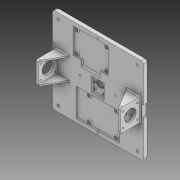
# Autodesk Inventor part: Topper
Saved by Autodesk Inventor 2020 (Build 240168000, 168)
## iProperties
Created: 2020-10-19
Part Number: Topper
Material: Generic
Document SubType Name: Modeling
Designer: DDeGo
Density: 1 g/cm^3
Appearance: Default
Author: DDeGo
Autodesk Inventor part; units mm, degrees
ref_plane "YZ Plane" through (0, 0, 0) normal (1, 0, 0) x (0, 1, 0)
ref_plane "XZ Plane" through (0, 0, 0) normal (0, 1, 0) x (-1, 0, 0)
sketch "Block1" plane through (0, 0, 0) normal (0, 0, 1) x (1, 0, 0)
  line L0 (-86.5, 19) -> (-20, 19) construction
  line L1 (-20, 19) -> (-20, 73.8) construction
  line L2 (-20, 73.8) -> (-86.5, 73.8) construction
  line L3 (-86.5, 73.8) -> (-86.5, 19) construction
  line L4 (-86.5, 19) -> (-20, 73.8) construction
  line L5 (-20, 19) -> (-86.5, 73.8) construction
  line L6 (-83, 22.15) -> (-23.5, 22.15) construction
  line L7 (-23.5, 22.15) -> (-23.5, 70.65) construction
  line L8 (-23.5, 70.65) -> (-83, 70.65) construction
  line L9 (-83, 70.65) -> (-83, 22.15) construction
  line L10 (-83, 22.15) -> (-23.5, 70.65) construction
  line L11 (-23.5, 22.15) -> (-83, 70.65) construction
  circle A0 centre (-23.5, 70.65) radius 1.35
  circle A1 centre (-83, 70.65) radius 1.35
  circle A2 centre (-23.5, 22.15) radius 1.35
  circle A3 centre (-83, 35) radius 1.35
  point P0 (-53.8698, 46.6979)
  point P1 (-53.25, 46.4)
  point P2 (-53.25, 46.4)
  dimension "d79" = 59.5
  dimension "d80" = 66.5
  dimension "d81" = 54.8
  dimension "d82" = 48.5
  dimension "d83" = 16
  dimension "d84" = 2.7
  measures "d79" distance of L7.end L8.end
  measures "d80" distance of L1.end L2.end
  measures "d81" distance of L0.end L1.end
  measures "d82" distance of L6.end L7.end
  measures "d83" distance from line of L0 A3.centre
  measures "d84" diameter of A3
sketch "Sketch1" plane through (0, 0, 0) normal (0, 0, 1) x (1, 0, 0)
  line L0 (-97.5, -92.5) -> (97.5, -92.5)
  line L1 (97.5, -92.5) -> (97.5, 92.5)
  line L2 (97.5, 92.5) -> (-97.5, 92.5)
  line L3 (-97.5, 92.5) -> (-97.5, -92.5)
  line L4 (-97.5, -92.5) -> (97.5, 92.5) construction
  line L5 (97.5, -92.5) -> (-97.5, 92.5) construction
  line L6 (85, -80) -> (-85, -80) construction
  line L7 (-85, -80) -> (-85, 80) construction
  line L8 (-85, 80) -> (85, 80) construction
  line L9 (85, 80) -> (85, -80) construction
  line L10 (85, -80) -> (-85, 80) construction
  line L11 (-85, -80) -> (85, 80) construction
  line L12 (-95.15, 90.15) -> (-74.85, 90.15)
  line L13 (-74.85, 90.15) -> (-74.85, 69.85)
  line L14 (-74.85, 69.85) -> (-95.15, 69.85)
  line L15 (-95.15, 69.85) -> (-95.15, 90.15)
  line L16 (-95.15, 90.15) -> (-74.85, 69.85) construction
  line L17 (-74.85, 90.15) -> (-95.15, 69.85) construction
  line L18 (95.15, 90.15) -> (74.85, 90.15)
  line L19 (74.85, 90.15) -> (74.85, 69.85)
  line L20 (74.85, 69.85) -> (95.15, 69.85)
  line L21 (95.15, 69.85) -> (95.15, 90.15)
  line L22 (95.15, 90.15) -> (74.85, 69.85) construction
  line L23 (74.85, 90.15) -> (95.15, 69.85) construction
  line L24 (95.15, -90.15) -> (74.85, -90.15)
  line L25 (74.85, -90.15) -> (74.85, -69.85)
  line L26 (74.85, -69.85) -> (95.15, -69.85)
  line L27 (95.15, -69.85) -> (95.15, -90.15)
  line L28 (95.15, -90.15) -> (74.85, -69.85) construction
  line L29 (74.85, -90.15) -> (95.15, -69.85) construction
  line L30 (-95.15, -90.15) -> (-74.85, -90.15)
  line L31 (-74.85, -90.15) -> (-74.85, -69.85)
  line L32 (-74.85, -69.85) -> (-95.15, -69.85)
  line L33 (-95.15, -69.85) -> (-95.15, -90.15)
  line L34 (-95.15, -90.15) -> (-74.85, -69.85) construction
  line L35 (-74.85, -90.15) -> (-95.15, -69.85) construction
  point P0 (0, 0)
  dimension "d0" = 195
  dimension "d2" = 170
  dimension "d23" = 185
  dimension "d24" = 160
  dimension "d113" = 20.3
  dimension "d114" = 20.3
  constraints: 72 end point, 12 midpoint, 12 parallel, 6 equal length, 6 horizontal, 6 perpendicular, 1 point on line
  measures "d0" distance of L1.end L2.end
  measures "d2" distance of L7.end L8.end
  measures "d23" distance of L0.end L1.end
  measures "d24" distance of L6.end L7.end
  measures "d113" distance of L12.start L12.end
  measures "d114" distance of L14.end L12.start
extrude "Extrusion1" add sketch "Sketch1" along normal blind 4
sketch "Sketch2" plane through (0, 0, 4) normal (0, 0, 1) x (1, 0, 0)
  line L0 (97.5, 92.5) -> (-97.5, 92.5) projected
  line L1 (97.5, -92.5) -> (-97.5, -92.5)
  line L2 (-97.5, -92.5) -> (-97.5, 92.5)
  line L3 (-97.5, 92.5) -> (97.5, 92.5)
  line L4 (97.5, 92.5) -> (97.5, -92.5)
  line L5 (97.5, -92.5) -> (-97.5, 92.5) construction
  line L6 (-97.5, -92.5) -> (97.5, 92.5) construction
  line L7 (-74.85, 69.85) -> (-95.15, 69.85) construction
  line L8 (-74.85, 90.15) -> (-74.85, 69.85) construction
  line L9 (-95.15, 69.85) -> (-74.85, 90.15) construction
  line L10 (74.85, 90.15) -> (95.15, 90.15) projected
  line L11 (95.15, 69.85) -> (74.85, 69.85) construction
  line L12 (74.85, 90.15) -> (95.15, 69.85) construction
  line L13 (74.85, -69.85) -> (95.15, -69.85) construction
  line L14 (74.85, -90.15) -> (74.85, -69.85) construction
  line L15 (95.15, -69.85) -> (74.85, -90.15) construction
  line L16 (-74.85, -90.15) -> (-95.15, -90.15) construction
  line L17 (-95.15, -90.15) -> (-95.15, -69.85) projected
  line L18 (-74.85, -90.15) -> (-95.15, -69.85) construction
  circle A0 centre (-85, 80) radius 2.75
  circle A1 centre (85, 80) radius 2.75
  circle A2 centre (85, -80) radius 2.75
  circle A3 centre (-85, -80) radius 2.75
  point P0 (0, 0)
  dimension "d7" = 5.5
  constraints: 16 end point, 4 centre point, 4 midpoint, 3 equal radius, 2 parallel, 1 horizontal, 1 perpendicular, 8 other
  measures "d7" diameter of A0
extrude "Extrusion2" add sketch "Sketch2" along normal blind 4
sketch "Sketch3" plane through (0, 0, 8) normal (0, 0, 1) x (1, 0, 0)
  line L0 (0, 0) -> (-96, 0) construction
  line L1 (0, 0) -> (96, 0) construction
  line L2 (-97.5, -12.5) -> (-94.5, -12.5)
  line L3 (-94.5, -12.5) -> (-94.5, 12.5)
  line L4 (-94.5, 12.5) -> (-97.5, 12.5)
  line L5 (-97.5, 12.5) -> (-97.5, -12.5)
  line L6 (-97.5, -12.5) -> (-94.5, 12.5) construction
  line L7 (-94.5, -12.5) -> (-97.5, 12.5) construction
  line L8 (94.5, -12.5) -> (97.5, -12.5)
  line L9 (97.5, -12.5) -> (97.5, 12.5)
  line L10 (97.5, 12.5) -> (94.5, 12.5)
  line L11 (94.5, 12.5) -> (94.5, -12.5)
  line L12 (94.5, -12.5) -> (97.5, 12.5) construction
  line L13 (97.5, -12.5) -> (94.5, 12.5) construction
  circle A0 centre (-85, 80) radius 2.75 projected
  line L14 (-85, 80) -> (-96, 0) construction
  circle A1 centre (85, 80) radius 2.75 projected
  line L15 (-97.5, 92.5) -> (-97.5, -92.5) projected
  dimension "d8" = 3
  dimension "d9" = 25
  constraints: 30 end point, 4 horizontal, 4 midpoint, 4 parallel, 3 equal length, 2 perpendicular, 1 point on line
  measures "d8" distance of L3.end L4.end
  measures "d9" distance of L2.end L3.end
extrude "Extrusion3" cut sketch "Sketch3" against normal through all contours L5 L4 L3 L2 | L11 L10 L9 L8
sketch "Sketch4" plane through (0, 0, 8) normal (0, 0, 1) x (1, 0, 0)
  line L0 (0, 0) -> (88.5, 0) construction
  line L1 (0, 0) -> (-88.5, 0) construction
  line L2 (-90.5, -21.15) -> (-86.5, -21.15)
  line L3 (-86.5, -21.15) -> (-86.5, 21.15)
  line L4 (-86.5, 21.15) -> (-90.5, 21.15)
  line L5 (-90.5, 21.15) -> (-90.5, -21.15)
  line L6 (-90.5, -21.15) -> (-86.5, 21.15) construction
  line L7 (-86.5, -21.15) -> (-90.5, 21.15) construction
  line L8 (86.5, -21.15) -> (90.5, -21.15)
  line L9 (90.5, -21.15) -> (90.5, 21.15)
  line L10 (90.5, 21.15) -> (86.5, 21.15)
  line L11 (86.5, 21.15) -> (86.5, -21.15)
  line L12 (86.5, -21.15) -> (90.5, 21.15) construction
  line L13 (90.5, -21.15) -> (86.5, 21.15) construction
  line L14 (-94.5, 12.5) -> (-94.5, -12.5) projected
  dimension "d13" = 42.3
  dimension "d14" = 4
  dimension "d22" = 8
  constraints: 28 end point, 4 horizontal, 4 midpoint, 4 parallel, 2 collinear, 2 perpendicular, 1 point on line
  measures "d13" distance of L2.end L3.end
  measures "d14" distance of L3.end L4.end
  measures "d22" distance between parallel lines of L14 L3
extrude "Extrusion4" add sketch "Sketch4" along normal blind 42.3
sketch "Sketch5" plane through (-90.5, -21.15, 8) normal (-1, 0, 0) x (0, 0, 1)
  line L0 (0, 0) -> (0, 42.3) projected
  line L1 (0, 0) -> (42.3, 0) projected
  line L2 (42.3, 42.3) -> (42.3, 0) projected
  line L3 (0, 42.3) -> (42.3, 42.3) projected
  line L4 (36.65, 5.65) -> (5.65, 5.65) construction
  line L5 (5.65, 5.65) -> (5.65, 36.65) construction
  line L6 (5.65, 36.65) -> (36.65, 36.65) construction
  line L7 (36.65, 36.65) -> (36.65, 5.65) construction
  line L8 (36.65, 36.65) -> (5.65, 5.65) construction
  circle A0 centre (36.65, 36.65) radius 1.75
  circle A1 centre (36.65, 5.65) radius 1.75
  circle A2 centre (21.15, 21.15) radius 12.5
  circle A3 centre (5.65, 5.65) radius 1.75
  circle A4 centre (5.65, 36.65) radius 1.75
  point P0 (-8, 21.15)
  dimension "d17" = 31
  dimension "d18" = 3.5
  dimension "d19" = 25
  constraints: 10 end point, 5 centre point, 4 coincident, 3 equal radius, 1 midpoint, 3 other
  measures "d17" distance of L6.end L4.start
  measures "d18" diameter of A1
  measures "d19" diameter of A2
extrude "Extrusion5" cut sketch "Sketch5" against normal through all contours A0 | A1 | A2 | A3 | A4
sketch "Sketch8" plane through (-90.5, -21.15, 8) normal (0, -1, 0) x (1, 0, 0)
  line L0 (4, 0) -> (0, 0) projected
  line L1 (4, 0) -> (4, 42.3) construction
  line L2 (0, 42.3) -> (4, 42.3) projected
  line L3 (0, 0) -> (0, 42.3) projected
  line L4 (181, 0) -> (177, 0) projected
  line L5 (181, 0) -> (181, 42.3) projected
  line L6 (177, 42.3) -> (181, 42.3) projected
  line L7 (177, 0) -> (177, 42.3) construction
  line L8 (4, 42.3) -> (28.4219, 0)
  line L9 (-7, 0) -> (188, 0) construction
  line L10 (4, 0) -> (28.4219, 0)
  line L11 (181, 42.3) -> (177, 42.3) projected
  line L12 (177, 42.3) -> (152.5781, 0)
  line L13 (152.5781, 0) -> (177, 0)
  point P0 (90.5, -8)
  dimension "d30" = 60
  dimension "d31" = 60
  constraints: 8 end point, 2 collinear, 2 point on line
  measures "d30" angle of L9 L8
  measures "d31" angle of L9 L12
extrude "Extrusion8" add sketch "Sketch8" along normal blind 3
mirror "Mirror1" about plane through (0, 0, 0) normal (0, 1, 0) of "Extrusion8"
ref_plane "Work Plane2" through (0, 0, 3.5) normal (0, 0, -1) x (-1, 0, 0)
sketch "Sketch6" plane through (0, 0, 8) normal (0, 0, 1) x (1, 0, 0)
  circle A0 centre (0, 0) radius 7
  dimension "d25" = 14
  constraints: 1 centre point, 1 coincident
  measures "d25" diameter of A0
extrude "Extrusion6" cut sketch "Sketch6" against normal through all
sketch "Sketch7" plane through (0, 0, 8) normal (0, 0, 1) x (1, 0, 0)
  circle A0 centre (0, 0) radius 7 projected
  line L0 (-13.5, 11) -> (13.5, 11)
  line L1 (13.5, 11) -> (13.5, -20)
  line L2 (13.5, -20) -> (-13.5, -20)
  line L3 (-13.5, -20) -> (-13.5, 11)
  dimension "d34" = 27
  dimension "d35" = 13.5
  dimension "d36" = 11
  dimension "d37" = 20
  constraints: 8 end point, 2 parallel, 1 horizontal, 1 perpendicular
  measures "d34" distance between parallel lines of L1 L3
  measures "d35" distance from line of L3 point (0, 0)
  measures "d36" distance from line of A0.centre L0
  measures "d37" distance from line of L2 A0.centre
extrude "Extrusion7" cut sketch "Sketch7" against normal up to surface (4.5 mm away)
sketch "Sketch9" plane through (-13.5, 11, 3.5) normal (0, 0, 1) x (1, 0, 0)
  circle A0 centre (23.75, -11) radius 1.2
  line L0 (23.75, -23.5) -> (23.75, -11) construction
  circle A1 centre (23.75, -23.5) radius 1.2
  line L1 (23.75, -11) -> (3.25, -11) construction
  circle A2 centre (3.25, -11) radius 1.2
  line L2 (3.25, -23.5) -> (23.75, -23.5) construction
  line L3 (3.25, -23.5) -> (23.75, -11) construction
  line L4 (3.25, -11) -> (3.25, -23.5) construction
  line L5 (23.75, -23.5) -> (3.25, -11) construction
  circle A3 centre (3.25, -23.5) radius 1.2
  line L6 (0, 0) -> (27, 0) projected
  line L7 (13.5, -17.25) -> (13.5, 0) construction
  line L8 (27, 0) -> (0, 0) projected
  point P0 (13.5, -11)
  dimension "d39" = 2.4
  dimension "d40" = 12.5
  dimension "d41" = 20.5
  constraints: 14 end point, 4 centre point, 4 coincident, 4 midpoint, 3 equal radius, 2 parallel, 1 horizontal, 1 perpendicular, 1 vertical
  measures "d39" diameter of A3
  measures "d40" distance of L1.end L2.start
  measures "d41" distance of L2.start L0.start
extrude "Extrusion9" cut sketch "Sketch9" against normal through all
fillet "Fillet1" radius 3 8 edges at (76.289, 24.15, 8) (76.289, -24.15, 8) (-76.289, 24.15, 8) (-76.289, -24.15, 8) (62.0781, 22.65, 8) (62.0781, -22.65, 8) (-62.0781, 22.65, 8) (-62.0781, -22.65, 8)
fillet "Fillet1" radius 2 2 edges at (-90.5, 0, 8) (90.5, 0, 8)
fillet "Fillet2" radius 5 4 edges at (-97.5, -92.5, 4) (97.5, -92.5, 4) (97.5, 92.5, 4) (-97.5, 92.5, 4)
sketch "Sketch10" plane through (0, 0, 8) normal (0, 0, 1) x (1, 0, 0)
  line L0 (22.5, 29.5) -> (22.5, 84.5)
  line L1 (22.5, 84.5) -> (-52.5, 84.5)
  line L2 (-52.5, 84.5) -> (-52.5, 29.5)
  line L3 (-52.5, 29.5) -> (22.5, 84.5) construction
  line L4 (22.5, 29.5) -> (-52.5, 84.5) construction
  line L5 (92.5, 92.5) -> (-92.5, 92.5) projected
  line L6 (-35, 19.5) -> (5, 19.5)
  line L7 (5, 19.5) -> (5, 29.5)
  line L8 (-35, 29.5) -> (-35, 19.5)
  line L9 (-35, 19.5) -> (5, 29.5) construction
  line L10 (5, 19.5) -> (-35, 29.5) construction
  line L11 (-52.5, 29.5) -> (-35, 29.5)
  line L12 (5, 29.5) -> (22.5, 29.5)
  line L13 (-15, 57) -> (-15, 19.5) construction
  point P0 (0, 0)
  point P1 (-15, 24.5)
  dimension "d48" = 55
  dimension "d49" = 75
  dimension "d50" = 8
  dimension "d60" = 40
  dimension "d61" = 10
  dimension "d116" = 15
  constraints: 26 end point, 4 midpoint, 4 parallel, 3 horizontal, 3 perpendicular, 2 collinear
  measures "d48" distance of L0.start L0.end
  measures "d49" distance of L0.end L1.end
  measures "d50" distance between parallel lines of L5 L1
  measures "d60" distance of L6.start L6.end
  measures "d61" distance of L6.end L7.end
  measures "d116" distance from line of point (0, 0) L13
extrude "Extrusion10" cut sketch "Sketch10" against normal blind 3
sketch "Sketch11" plane through (0, 0, 5) normal (0, 0, 1) x (1, 0, 0)
  line L0 (-52.5, 84.5) -> (22.5, 84.5) projected
  line L1 (-35, 29.5) -> (-52.5, 29.5) projected
  line L2 (-52.5, 84.5) -> (22.5, 29.5) construction
  line L3 (-47, 34.875) -> (17, 34.875) construction
  line L4 (17, 34.875) -> (17, 79.125) construction
  line L5 (17, 79.125) -> (-47, 79.125) construction
  line L6 (-47, 79.125) -> (-47, 34.875) construction
  line L7 (-47, 34.875) -> (17, 79.125) construction
  line L8 (17, 34.875) -> (-47, 79.125) construction
  circle A0 centre (-47, 34.875) radius 1.25
  circle A1 centre (17, 34.875) radius 1.25
  circle A2 centre (-47, 79.125) radius 1.25
  circle A3 centre (17, 79.125) radius 1.25
  circle A4 centre (-47, 79.125) radius 3
  circle A5 centre (-47, 34.875) radius 3
  circle A6 centre (17, 79.125) radius 3
  circle A7 centre (17, 34.875) radius 3
  point P0 (0, 0)
  point P1 (-15, 57)
  dimension "d53" = 2.5
  dimension "d54" = 6
  dimension "d103" = 44.25
  dimension "d104" = 64
  constraints: 14 end point, 9 coincident, 8 centre point, 6 equal radius, 3 midpoint, 2 parallel, 1 horizontal, 1 perpendicular
  measures "d53" diameter of A2
  measures "d54" diameter of A4
  measures "d103" distance of L5.end L3.start
  measures "d104" distance of L3.start L3.end
extrude "Extrusion11" add sketch "Sketch11" along normal blind 3
sketch "Sketch12" plane through (0, 0, 8) normal (0, 0, 1) x (1, 0, 0)
  line L0 (0, 0) -> (0, -54.5) construction
  line L1 (-46, -24.5) -> (46, -24.5)
  line L2 (46, -24.5) -> (46, -84.5)
  line L3 (46, -84.5) -> (-46, -84.5)
  line L4 (-46, -84.5) -> (-46, -24.5)
  line L5 (-46, -24.5) -> (46, -84.5) construction
  line L6 (46, -24.5) -> (-46, -84.5) construction
  line L7 (-92.5, -92.5) -> (92.5, -92.5) projected
  dimension "d62" = 8
  dimension "d85" = 92
  dimension "d86" = 60
  constraints: 14 end point, 2 midpoint, 2 parallel, 1 horizontal, 1 perpendicular, 1 vertical
  measures "d62" distance between parallel lines of L7 L3
  measures "d85" distance of L2.end L3.end
  measures "d86" distance of L1.end L2.end
extrude "Extrusion12" cut sketch "Sketch12" against normal up to surface (3 mm away)
sketch "Sketch13" plane through (0, 0, 8) normal (0, 0, 1) x (1, 0, 0)
  circle A0 centre (-38, 0) radius 1.45 projected
  circle A1 centre (0, 88) radius 1.45 projected
  circle A2 centre (93, 32) radius 1.45 projected
  circle A3 centre (-93, 32) radius 1.45 projected
  circle A4 centre (38, 0) radius 1.45 projected
  circle A5 centre (0, -88) radius 1.45 projected
  circle A6 centre (93, -32) radius 1.45 projected
  circle A7 centre (-93, -32) radius 1.45 projected
  point P0 (0, 0)
extrude "Extrusion13" cut sketch "Sketch13" against normal through all
sketch "Sketch14" plane through (0, 0, 0) normal (0, 0, -1) x (-1, 0, 0)
  circle A0 centre (93, -32) radius 1.45 construction
  circle A1 centre (0, -88) radius 1.45 construction
  circle A2 centre (-93, -32) radius 1.45 construction
  circle A3 centre (-93, 32) radius 1.45 construction
  circle A4 centre (0, 88) radius 1.45 construction
  circle A5 centre (93, 32) radius 1.45 construction
  circle A6 centre (93, -32) radius 1.75
  circle A7 centre (93, 32) radius 1.45 construction
  circle A8 centre (93, 32) radius 1.75
  circle A9 centre (0, -88) radius 1.75
  circle A10 centre (-93, 32) radius 1.45 construction
  circle A11 centre (-93, 32) radius 1.75
  circle A12 centre (-93, -32) radius 1.45 construction
  circle A13 centre (-93, -32) radius 1.75
  circle A14 centre (0, 88) radius 1.75
  circle A15 centre (38, 0) radius 1.45 construction
  circle A16 centre (38, 0) radius 1.75
  circle A17 centre (-38, 0) radius 1.45 construction
  circle A18 centre (-38, 0) radius 1.75
  point P0 (0, 0)
  dimension "d67" = 3.5
  constraints: 8 centre point, 8 coincident, 7 equal radius
  measures "d67" diameter of A11
extrude "Extrusion14" cut sketch "Sketch14" against normal through all
sketch "Sketch15" plane through (0, 0, 0) normal (0, 0, -1) x (-1, 0, 0)
  circle A0 centre (93, -32) radius 1.75 construction
  circle A1 centre (93, 32) radius 1.75 construction
  circle A2 centre (0, 88) radius 1.75 construction
  circle A3 centre (-93, 32) radius 1.75 construction
  circle A4 centre (-93, -32) radius 1.75 construction
  circle A5 centre (0, -88) radius 1.75 construction
  circle A6 centre (38, 0) radius 1.75 construction
  circle A7 centre (-38, 0) radius 1.75 construction
  circle A8 centre (93, -32) radius 3
  circle A9 centre (38, 0) radius 3
  circle A10 centre (-38, 0) radius 1.75 construction
  circle A11 centre (-38, 0) radius 3
  circle A12 centre (-93, -32) radius 3
  circle A13 centre (93, 32) radius 3
  circle A14 centre (0, 88) radius 3
  circle A15 centre (0, -88) radius 3
  circle A16 centre (-93, 32) radius 3
  point P0 (0, 0)
  dimension "d70" = 6
  constraints: 8 centre point, 8 coincident, 7 equal radius
  measures "d70" diameter of A15
extrude "Extrusion15" cut sketch "Sketch15" against normal blind 4
sketch "Sketch16" plane through (-13.5, -20, 3.5) normal (0, 0, 1) x (1, 0, 0)
  circle A0 centre (3.25, 20) radius 1.2 projected
  circle A1 centre (23.75, 20) radius 1.2 projected
  circle A2 centre (23.75, 7.5) radius 1.2 projected
  circle A3 centre (3.25, 7.5) radius 1.2 projected
  circle A4 centre (3.25, 20) radius 1.2 projected
  circle A5 centre (3.25, 20) radius 2.5
  circle A6 centre (23.75, 20) radius 1.2 projected
  circle A7 centre (23.75, 20) radius 2.5
  circle A8 centre (23.75, 7.5) radius 1.2 projected
  circle A9 centre (23.75, 7.5) radius 2.5
  circle A10 centre (3.25, 7.5) radius 2.5
  point P0 (13.5, 20)
  dimension "d73" = 5
  constraints: 4 centre point, 4 coincident, 3 equal radius
  measures "d73" diameter of A5
extrude "Extrusion16" add sketch "Sketch16" along normal blind 3
chamfer "Chamfer2" distance 2.5 angle 45 1 edges at (-7, 0, 0)
sketch "Sketch17" plane through (-46, -24.5, 5) normal (0, 0, 1) x (1, 0, 0)
  line L0 (2, -2) -> (87, -2) construction
  line L1 (87, -2) -> (87, -58) construction
  line L2 (87, -58) -> (2, -58) construction
  line L3 (2, -58) -> (2, -2) construction
  line L4 (25.5, -5.5) -> (83.5, -5.5) construction
  line L5 (83.5, -5.5) -> (83.5, -54.5) construction
  line L6 (83.5, -54.5) -> (25.5, -54.5) construction
  line L7 (25.5, -54.5) -> (25.5, -5.5) construction
  line L8 (0, -60) -> (0, 0) projected
  line L9 (0, 0) -> (92, 0) projected
  circle A0 centre (25.5, -5.5) radius 1.25
  circle A1 centre (83.5, -5.5) radius 1.25
  circle A2 centre (83.5, -54.5) radius 1.25
  circle A3 centre (25.5, -54.5) radius 1.25
  circle A4 centre (25.5, -54.5) radius 3
  circle A5 centre (25.5, -5.5) radius 3
  circle A6 centre (83.5, -5.5) radius 3
  circle A7 centre (83.5, -54.5) radius 3
  point P0 (46, 24.5)
  dimension "d87" = 56
  dimension "d88" = 85
  dimension "d89" = 2
  dimension "d90" = 2
  dimension "d91" = 49
  dimension "d92" = 58
  dimension "d94" = 3.5
  dimension "d95" = 3.5
  dimension "d96" = 2.5
  dimension "d97" = 6
  dimension "d117" = 3.5
  constraints: 16 end point, 8 centre point, 8 coincident, 6 equal radius, 4 parallel, 2 horizontal, 2 perpendicular
  measures "d87" distance of L2.end L0.start
  measures "d88" distance of L0.start L0.end
  measures "d89" distance between parallel lines of L8 L3
  measures "d90" distance between parallel lines of L9 L0
  measures "d91" distance of L6.end L4.start
  measures "d92" distance of L4.start L4.end
  measures "d94" distance between parallel lines of L2 L6
  measures "d95" distance between parallel lines of L0 L4
  measures "d96" diameter of A0
  measures "d97" diameter of A5
  measures "d117" distance between parallel lines of L1 L5
extrude "Extrusion17" add sketch "Sketch17" along normal up to surface (3 mm away)
chamfer "Chamfer3" distance 0.5 angle 45 12 edges at (-50, 79.125, 8) (-50, 34.875, 8) (14, 34.875, 8) (14, 79.125, 8) (-12.75, 0, 6.5) (7.75, 0, 6.5) (7.75, -12.5, 6.5) (-12.75, -12.5, 6.5) (-23.5, -30, 8) (34.5, -30, 8) (34.5, -79, 8) (-23.5, -79, 8)
chamfer "Chamfer4" distance 3 angle 45 1 edges at (-15, 19.5, 8)
fillet "Fillet3" radius 4 4 edges at (-88.5, 24.15, 50.3) (-88.5, -24.15, 50.3) (88.5, -24.15, 50.3) (88.5, 24.15, 50.3)
sketch "Sketch18" plane through (0, 0, 8) normal (0, 0, 1) x (1, 0, 0)
  line L0 (41, -64.5) -> (51, -64.5)
  line L1 (51, -64.5) -> (51, -44.5)
  line L2 (51, -44.5) -> (41, -44.5)
  line L3 (41, -44.5) -> (41, -64.5)
  line L4 (41, -64.5) -> (51, -44.5) construction
  line L5 (51, -64.5) -> (41, -44.5) construction
  line L6 (46, -24.5) -> (46, -84.5) projected
  point P0 (0, 0)
  point P1 (46, -54.5)
  dimension "d109" = 10
  dimension "d110" = 20
  constraints: 12 end point, 3 midpoint, 2 parallel, 1 horizontal, 1 perpendicular
  measures "d109" distance of L1.end L2.end
  measures "d110" distance of L0.end L1.end
extrude "Extrusion18" cut sketch "Sketch18" against normal up to surface (3 mm away)
fillet "Fillet4" radius 2 8 edges at (-50, 79.125, 5) (14, 79.125, 5) (-50, 34.875, 5) (14, 34.875, 5) (-23.5, -30, 5) (34.5, -30, 5) (34.5, -79, 5) (-23.5, -79, 5)
ref_plane "Work Plane1" through (0, 0, 0) normal (0, 1, 0) x (-1, 0, 0)
equation "\"d35\" = 0.5 * d34"
body "Solid1"
